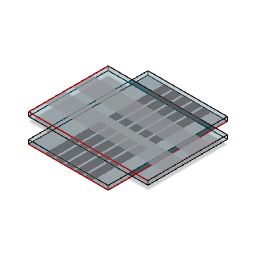
Assembly (Autodesk Fusion 360 archive; units mm, degrees)
design "TCA Test Structure"
Autodesk Fusion 360 part; units mm, degrees
sketch "Sketch1" plane through (0, 0, 0) normal (0, 1, 0) x (1, 0, 0)
  line L0 (10, -15) -> (-10, -15)
  line L1 (-10, -15) -> (-10, 15)
  line L2 (-10, 15) -> (10, 15)
  line L3 (10, 15) -> (10, -15)
  line L4 (10, -15) -> (-10, 15) construction
  line L5 (-10, -15) -> (10, 15) construction
  dimension "d1" = 20
  dimension "d2" = 30
  constraint perpendicular L0 L1
  constraint parallel L0 L2
  constraint parallel L1 L3
  constraint horizontal L0
  constraint coincident L4 origin
  constraint coincident L5 origin
  measures "d1" distance of L1.end L2.end
  measures "d2" distance of L0.end L1.end
extrude "Extrude1" add sketch "Sketch1" along normal blind 1
sketch "Sketch2" plane through (0, 1, 0) normal (0, 1, 0) x (-1, 0, 0)
  line L0 (-10, -15) -> (10, -15)
  line L1 (10, -15) -> (10, 15)
  line L2 (10, 15) -> (-10, 15)
  line L3 (-10, 15) -> (-10, -15)
  line L4 (-10, 10) -> (10, 10)
  line L5 (10, 10) -> (10, -10)
  line L6 (10, -10) -> (-10, -10)
  line L7 (-10, -10) -> (-10, 10)
  line L8 (-10, 10) -> (10, -10) construction
  line L9 (10, 10) -> (-10, -10) construction
  dimension "d5" = 20
  constraint perpendicular L4 L5
  constraint parallel L4 L6
  constraint parallel L5 L7
  constraint horizontal L4
  constraint coincident L3 L4.start
  constraint coincident L8 origin
  constraint coincident L9 origin
  measures "d5" distance of L4.end L5.end
extrude "Extrude2" add sketch "Sketch2" along normal blind 0.04 contours L1 L3 L4 L5 L6 L7
sketch "Sketch3" plane through (0, 1.04, 0) normal (0, 1, 0) x (-1, 0, 0)
  line L0 (-10, -10) -> (10, -10)
  line L1 (10, -10) -> (10, 10)
  line L2 (10, 10) -> (-10, 10)
  line L3 (-10, 10) -> (-10, -10)
  line L4 (-15, 10) -> (15, 10)
  line L5 (15, 10) -> (15, -10)
  line L6 (15, -10) -> (-15, -10)
  line L7 (-15, -10) -> (-15, 10)
  line L8 (-15, 10) -> (15, -10) construction
  line L9 (15, 10) -> (-15, -10) construction
  dimension "d8" = 30
  dimension "d9" = 20
  constraint perpendicular L4 L5
  constraint parallel L4 L6
  constraint parallel L5 L7
  constraint horizontal L4
  constraint coincident L8 origin
  constraint coincident L9 origin
  measures "d8" distance of L5.end L6.end
  measures "d9" distance of L4.end L5.end
extrude "Extrude3" add sketch "Sketch3" along normal blind 1

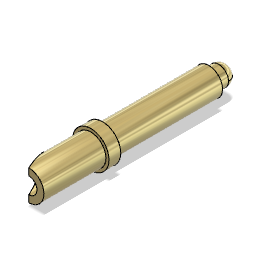
design "Pins"
Autodesk Fusion 360 part; units mm, degrees
sketch "Sketch2" plane through (0, 0, 0) normal (0, 1, 0) x (1, 0, 0)
  line L0 (0, 0) -> (0, 10.81)
  line L1 (0, 10.81) -> (0.535, 10.81)
  line L2 (0.535, 10.81) -> (0.535, 9.8047)
  line L3 (0, 9.81) -> (0.75, 9.81)
  line L4 (0.75, 9.81) -> (0.75, 4.02)
  line L5 (0, 4.02) -> (0.99, 4.02)
  line L6 (0.99, 4.02) -> (0.99, 3.38)
  line L7 (0, 3.38) -> (0.825, 3.38)
  line L8 (0.99, 3.38) -> (0.825, 3.38)
  line L9 (0.825, 3.38) -> (0.825, 0)
  line L10 (0.825, 0) -> (0, 0)
  line L11 (0.535, 10.11) -> (0.535, 9.81)
  spline S0 degree 5 poles (0, 10.81) (0.0206, 10.81) (0.0609, 10.8092) (0.1188, 10.8056) (0.1908, 10.7959) (0.2714, 10.7751) (0.3418, 10.7448) (0.4011, 10.7042) (0.4489, 10.6529) (0.4856, 10.5913) (0.5121, 10.5201) (0.5256, 10.4562) (0.5318, 10.4045) (0.5342, 10.3684) (0.535, 10.35) knots 0 0 0 0 0 0 0.1 0.2 0.3 0.4 0.5 0.6 0.7 0.8 0.9 1 1 1 1 1 1
  point P0 (0.4, 10.7)
  dimension "d2" = 10.81
  dimension "d3" = 0.535
  dimension "d4" = 0.7
  dimension "d5" = 0.75
  dimension "d6" = 5.79
  dimension "d7" = 0.99
  dimension "d8" = 0.64
  dimension "d9" = 0.825
  dimension "d10" = 3.38
  constraint coincident L0.start L10.end
  constraint vertical L0
  constraint perpendicular L0 L1
  constraint perpendicular L1 L2
  constraint coincident L0 L3.start
  constraint perpendicular L0 L3
  constraint perpendicular L3 L4
  constraint coincident L0 L5.start
  constraint perpendicular L4 L5
  constraint perpendicular L5 L6
  constraint coincident L0 L7.start
  constraint perpendicular L6 L7
  constraint perpendicular L6 L8
  constraint perpendicular L8 L9
  constraint perpendicular L0 L10
  constraint coincident L3 L11.end
  constraint perpendicular L3 L11
  constraint coincident L2 S0.end
  measures "d2" distance of L0.start L0.end
  measures "d3" distance of L0.end L1.end
  measures "d4" distance of L1.end L11.start
  measures "d5" distance of L3.start L3.end
  measures "d6" distance of L3.end L4.end
  measures "d7" distance of L5.start L5.end
  measures "d8" distance of L5.end L6.end
  measures "d9" distance of L7.start L7.end
  measures "d10" distance of L7.end L9.end
revolve "Revolve1" add sketch "Sketch2" angle 360 about axis through (0, 0, 1.75) along (0, 0, 1) contours L0 L7 L9 L10 | L0 L5 L6 L7 L8 | L0 L3 L4 L5 | L0 L2 L3 L11 S0 makes body 1
sketch "Sketch3" plane through (0, 0, 0) normal (0, 0, 1) x (1, 0, 0)
  circle A0 centre (0, 0) radius 0.825
  circle A1 centre (0, 0) radius 0.445
  dimension "d12" = 0.89
  constraint concentric A0 A1
  measures "d12" diameter of A1
extrude "Extrude1" cut sketch "Sketch3" against normal blind 4.57 contours A1 bodies 1
sketch "Sketch4" plane through (0, 0, 0) normal (0, 1, 0) x (1, 0, 0)
  line L0 (0, 0) -> (0, 2.26)
  line L1 (0, 2.26) -> (-1, 2.26)
  line L2 (-1, 2.26) -> (0, 0)
  line L3 (-1, 0) -> (-1, 2.26)
  line L4 (-1, 0) -> (0, 0)
  dimension "d15" = 2.26
  constraint coincident L0.start L2.end
  constraint vertical L0
  constraint perpendicular L0 L1
  constraint perpendicular L1 L3
  constraint perpendicular L0 L4
  measures "d15" distance of L0.start L0.end
extrude "Extrude2" cut sketch "Sketch4" along normal blind 1.5 and the other way blind 1.5 contours L2 L3 L4 bodies 1
copy_body "Body->Comp1" bodies 1 removing the originals makes body 2 in component "SolderPin"
component "SolderPin" placed x (1, 0, 0) y (0, 1, 0) z (0, 0, 1) at (0, 0, 0)
equation "d2 = 1 mm + 6.43 mm + 3.38 mm"
equation "d3 = ( 1.07 / 2 ) * 1 mm"
equation "d5 = ( 1.5 / 2 ) * 1 mm"
equation "d6 = 6.43 mm - 0.64 mm"
equation "d7 = ( 1.98 / 2 ) * 1 mm"
equation "d9 = ( 1.65 / 2 ) * 1 mm"
